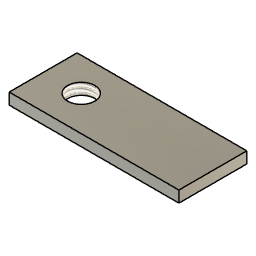
patient_side v1 (Autodesk Fusion 360 design; units mm, degrees)
Autodesk Fusion 360 part; units mm, degrees
sketch "Sketch1" plane through (0, 0, 0) normal (0, 0, 1) x (1, 0, 0)
  line L0 (0, 0) -> (75, 0)
  line L1 (75, 0) -> (75, 30)
  line L2 (75, 30) -> (0, 30)
  line L3 (0, 30) -> (0, 0)
  constraint horizontal L0
  constraint vertical L1
  constraint horizontal L2
  constraint vertical L3
  constraint coincident L0.start L3.end
extrude "Extrude1" add sketch "Sketch1" along normal blind 5
hole "Hole1" at (16.3939, 15.4301, 5) direction (0, 0, -1) diameter 12.023 depth 10 tip angle 180
thread "Thread1" "ISO Metric profile 14.0 M14x2 M14x2 6H" thread offset 0 thread depth 7.4
